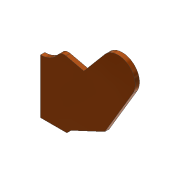
# Autodesk Inventor part: HIP_TOPFRAME2
Saved by Autodesk Inventor 2019.4 (Build 234330000, 330)
## iProperties
Created: 2019-11-06
Part Number: HIP_TOPFRAME2
Material: 一般
Document SubType Name: Modeling
Designer: y6tada
Density: 1 g/cm^3
Appearance: 滑らか - 淡いオレンジ
Author: y6tada
Autodesk Inventor part; units mm, degrees
ref_plane "YZ Plane" through (0, 0, 0) normal (1, 0, 0) x (0, 1, 0)
ref_plane "XZ Plane" through (0, 0, 0) normal (0, 1, 0) x (-1, 0, 0)
ref_plane "XY Plane" through (0, 0, 0) normal (0, 0, 1) x (1, 0, 0)
sketch "スケッチ1" plane through (0, 0, 0) normal (0, 0, 1) x (0, 1, 0)
  circle A0 centre (12, 0) radius 4 construction
  arc A1 (2, 0) -> (6.1183, -8.0874) centre (12, 0) ccw
  arc A2 (7.5078, -11.8161) -> (6.1183, -8.0874) centre (4, -11) ccw
  line L0 (-23.25, 12.25) -> (-23.25, -12.25) construction
  line L1 (-23.25, -12.25) -> (-21.25, -14.25) construction
  line L2 (-21.25, -14.25) -> (21.25, -14.25) construction
  line L3 (0, 0) -> (2, 0)
  line L4 (0, 0) -> (-23.25, 0)
  line L5 (-23.25, 0) -> (-23.25, -12.25)
  line L6 (-23.25, -12.25) -> (-21.25, -14.25)
  line L7 (-21.25, -14.25) -> (-13.9525, -29.8743)
  line L8 (-13.9525, -29.8743) -> (7.911, -42.876)
  line L9 (7.5078, -11.8161) -> (5.5688, -20.1499)
  line L10 (5.5688, -20.1499) -> (17.1455, -29.8743)
  line L11 (2, 0) -> (12, 0) construction
  circle A3 centre (4, -11) radius 1.25 construction
  arc A4 (7.911, -42.876) -> (17.1455, -29.8743) centre (12, -36) ccw
  circle A5 centre (-20, -11) radius 1.25 construction
  line L12 (12, 0) -> (12, -36) construction
  dimension "d0" = 10
  dimension "d3" = 36
  dimension "d4" = 8
  constraints: 20 end point, 6 point on circle, 4 tangent, 3 centre point, 3 coincident, 2 collinear, 2 concentric, 2 horizontal, 1 midpoint, 1 vertical
  measures "d0" radius of A1
  measures "d3" distance of L12.start L12.end
  measures "d4" radius of A4
extrude "押し出し1" add sketch "スケッチ1" along normal blind 2
